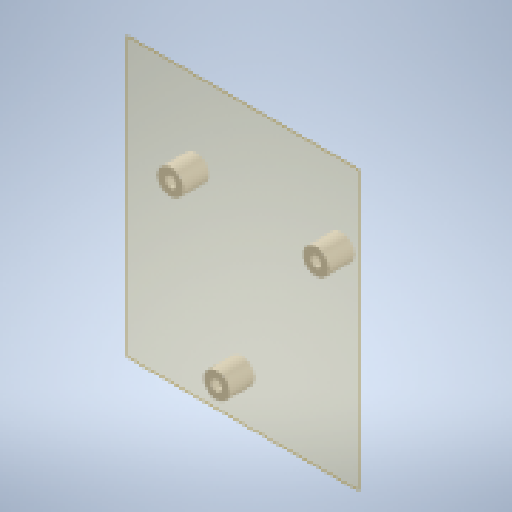
# Autodesk Inventor part: gyrholder
Saved by Autodesk Inventor 2023 (Build 270158000, 158)
## iProperties
Created: 2023-11-07
Part Number: gyrholder
Material: Générique
Document SubType Name: Modeling
Designer: eleves
Density: 1 g/cm^3
Appearance: Par défaut
Author: eleves
Autodesk Inventor part; units mm, degrees
ref_plane "YZ Plane" through (0, 0, 0) normal (1, 0, 0) x (0, 1, 0)
ref_plane "XZ Plane" through (0, 0, 0) normal (0, 1, 0) x (-1, 0, 0)
ref_plane "XY Plane" through (0, 0, 0) normal (0, 0, 1) x (1, 0, 0)
ref_plane "Plan de construction1" through (0, 0, 0) normal (0, 0, 1) x (1, 0, 0)
sketch "Esquisse1" plane through (0, 0, 0) normal (0, 0, 1) x (1, 0, 0)
  circle A0 centre (43.13, -2.93) radius 1.738 projected
  circle A1 centre (-5.13, -4.2) radius 1.738 projected
  circle A2 centre (10.11, -55) radius 1.738 projected
  circle A3 centre (-5.13, -4.2) radius 4.238
  circle A4 centre (43.13, -2.93) radius 4.238
  circle A5 centre (10.11, -55) radius 4.238
  point P0 (0, 0)
  dimension "d0" = 2.5
  dimension "d1" = 2.5
  dimension "d2" = 2.5
  constraints: 3 centre point
  measures "d0" radial gap between concentric circles of A1 A3
  measures "d1" radial gap between concentric circles of A2 A5
  measures "d2" radial gap between concentric circles of A0 A4
ref_plane "Plan de construction2" through (-15.898, -57.398, -8.5) normal (0, 0, 1) x (1, 0, 0)
extrude "Extrusion1" add sketch "Esquisse1" against normal up to surface (8.5 mm away)
sketch "Esquisse3" plane through (43.13, -2.93, 0) normal (0, 0, 1) x (1, 0, 0)
  circle A0 centre (0, 0) radius 4.238 projected
  circle A1 centre (0, 0) radius 1.738 projected
  circle A2 centre (-48.26, -1.27) radius 4.238 projected
  circle A3 centre (-48.26, -1.27) radius 1.738 projected
  circle A4 centre (-33.02, -52.07) radius 4.238 projected
  circle A5 centre (-33.02, -52.07) radius 1.738 projected
  point P0 (-43.13, 2.93)
extrude "Extrusion2" add sketch "Esquisse3" along normal blind 5
sketch "Esquisse4" plane through (43.13, -2.93, 5) normal (0, 0, 1) x (1, 0, 0)
  circle A0 centre (-48.26, -1.27) radius 1.738 projected
  circle A1 centre (-33.02, -52.07) radius 1.738 projected
  line L0 (-48.26, -1.27) -> (-33.02, -52.07) construction
  line L1 (-54.007, -2.9941) -> (-38.767, -53.7941)
  line L2 (-27.273, -50.3459) -> (-42.513, 0.4541)
  arc A2 (-42.513, 0.4541) -> (-54.007, -2.9941) centre (-48.26, -1.27) ccw
  arc A3 (-38.767, -53.7941) -> (-27.273, -50.3459) centre (-33.02, -52.07) ccw
  line L3 (-48.26, -1.27) -> (0, 0) construction
  line L4 (-48.1022, -7.2679) -> (0.1578, -5.9979)
  line L5 (-0.1578, 5.9979) -> (-48.4178, 4.7279)
  arc A4 (-48.4178, 4.7279) -> (-48.1022, -7.2679) centre (-48.26, -1.27) ccw
  arc A5 (0.1578, -5.9979) -> (-0.1578, 5.9979) centre (0, 0) ccw
  circle A6 centre (-33.02, -52.07) radius 4.238 projected
  line L6 (-33.02, -52.07) -> (0, 0) construction
  line L7 (-27.9529, -55.2833) -> (5.0671, -3.2133)
  line L8 (-5.0671, 3.2133) -> (-38.0871, -48.8567)
  arc A7 (-38.0871, -48.8567) -> (-27.9529, -55.2833) centre (-33.02, -52.07) ccw
  arc A8 (5.0671, -3.2133) -> (-5.0671, 3.2133) centre (0, 0) ccw
  circle A9 centre (0, 0) radius 4.238 projected
  circle A10 centre (0, 0) radius 1.738 projected
  point P0 (-43.13, 2.93)
  point P1 (-40.64, -26.67)
  point P2 (-24.13, -0.635)
  point P3 (-16.51, -26.035)
  point P4 (5.0671, -3.2133)
  point P5 (-11.0961, -6.2941)
  point P6 (-31.0492, -37.7586)
  point P7 (-40.2584, -7.0615)
  dimension "d7" = 12
  dimension "d8" = 12
  dimension "d9" = 12
  constraints: 24 end point, 12 point on circle, 12 tangent, 6 centre point, 3 midpoint, 3 parallel
  measures "d7" distance between parallel lines of L1 L2
  measures "d8" distance between parallel lines of L7 L8
  measures "d9" distance between parallel lines of L4 L5
extrude "Extrusion3" add sketch "Esquisse4" along normal blind 5 contours A4 L4 L2 L8 A7 L1 | A2 L2 L4 A4 | A7 L8 L2 A3 | L5 A8 L8 L4 L2 A2 | A3 L2 L8 L4 A5 L7 | A5 L4 L8 A8 | A6 | A9
sketch "Esquisse5" plane through (43.13, -2.93, 10) normal (0, 0, 1) x (1, 0, 0)
  line L0 (2.9, 1.6743) -> (2.9, -1.6743)
  line L1 (2.9, -1.6743) -> (0, -3.3486)
  line L2 (0, -3.3486) -> (-2.9, -1.6743)
  line L3 (-2.9, -1.6743) -> (-2.9, 1.6743)
  line L4 (-2.9, 1.6743) -> (0, 3.3486)
  line L5 (0, 3.3486) -> (2.9, 1.6743)
  circle A0 centre (-48.26, -1.27) radius 1.738 projected
  line L6 (-45.36, -2.9443) -> (-48.26, -4.6186)
  line L7 (-48.26, -4.6186) -> (-51.16, -2.9443)
  line L8 (-51.16, -2.9443) -> (-51.16, 0.4043)
  line L9 (-51.16, 0.4043) -> (-48.26, 2.0786)
  line L10 (-48.26, 2.0786) -> (-45.36, 0.4043)
  line L11 (-45.36, 0.4043) -> (-45.36, -2.9443)
  circle A1 centre (-33.02, -52.07) radius 1.738 projected
  line L12 (-33.02, -48.7214) -> (-30.12, -50.3957)
  line L13 (-30.12, -50.3957) -> (-30.12, -53.7443)
  line L14 (-30.12, -53.7443) -> (-33.02, -55.4186)
  line L15 (-33.02, -55.4186) -> (-35.92, -53.7443)
  line L16 (-35.92, -53.7443) -> (-35.92, -50.3957)
  line L17 (-35.92, -50.3957) -> (-33.02, -48.7214)
  point P0 (-43.13, 2.93)
  point P1 (0, 0)
  point P2 (0, 0)
  dimension "d12" = 5.8
  dimension "d13" = 5.8
  dimension "d14" = 5.8
  constraints: 36 end point, 3 coincident, 3 vertical, 40 other
  measures "d12" distance between parallel lines of L13 L16
  measures "d13" distance between parallel lines of L7 L10
  measures "d14" distance between parallel lines of L1 L4
extrude "Extrusion4" cut sketch "Esquisse5" against normal blind 2.5 contours L0 L1 L2 L3 L4 L5 | A0 | L6 L7 L8 L9 L10 L11 | A1 | L12 L13 L14 L15 L16 L17
sketch "Esquisse6" plane through (43.13, -2.93, 10) normal (0, 0, 1) x (1, 0, 0)
  point P0 (-43.13, 2.93)
